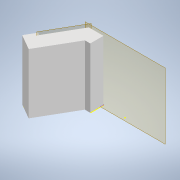
# Autodesk Inventor part: Задние_кресла
Saved by Autodesk Inventor 2021.2 (Build 252289000, 289)
## iProperties
Created: 2021-10-13
Part Number: Задние_кресла
Material: Типовые
Document SubType Name: Modeling
Designer: Surflay
Density: 1 g/cm^3
Appearance: По умолчанию
Author: Surflay
Autodesk Inventor part; units mm, degrees
ref_plane "YZ Plane" through (0, 0, 0) normal (1, 0, 0) x (0, 1, 0)
ref_plane "XZ Plane" through (0, 0, 0) normal (0, 1, 0) x (-1, 0, 0)
ref_plane "XY Plane" through (0, 0, 0) normal (0, 0, 1) x (1, 0, 0)
ref_plane "РабПлоскость1" through (0, 0, 0) normal (0, 0, 1) x (1, 0, 0)
sketch "Эскиз1" plane through (0, 0, 0) normal (0, 0, 1) x (1, 0, 0)
  line L0 (-185, -102) -> (-185, 102) projected
  line L1 (-123.5, -102) -> (-185, -102) projected
  line L2 (-123.5, 102) -> (-123.5, -102) projected
  line L3 (-185, 102) -> (-123.5, 102) projected
  line L4 (-123.5, 102) -> (-123.5, -102) projected
  line L5 (-123.5, -102) -> (123.5, -102) projected
  line L6 (123.5, -102) -> (123.5, -100.4305) projected
  line L7 (123.5, -100.4305) -> (123.5, 102) projected
  line L8 (123.5, 102) -> (-123.5, 102) projected
  line L9 (-123.5, -102) -> (-73.5, -102)
  line L10 (-73.5, -102) -> (-73.5, 102)
  line L11 (-73.5, 102) -> (-123.5, 102)
  line L12 (-123.5, 102) -> (-123.5, -102)
  point P0 (0, 0)
  dimension "d0" = 50
  constraints: 8 end point, 2 parallel, 1 horizontal, 1 perpendicular, 1 point on line
  measures "d0" distance of L11.end L10.end
extrude "Выдавливание1" add sketch "Эскиз1" along normal blind 45 contours L2 L8 L10 L5
ref_plane "РабПлоскость2" through (-154.25, 0, 53.2606) normal (0.866, 0, 0.5) x (0, 1, 0)
sketch "Эскиз2" plane through (-154.25, 0, 53.2606) normal (0.866, 0, 0.5) x (0, 1, 0)
  line L0 (-102, 61.5) -> (102, 61.5) projected
  line L1 (-102, -61.5) -> (-102, 61.5) projected
  line L2 (102, -61.5) -> (-102, -61.5) projected
  line L3 (102, 61.5) -> (102, -61.5) projected
  line L4 (102, -61.5) -> (-102, -61.5) projected
  line L5 (-102, -61.5) -> (-102, -185) projected
  line L6 (-102, -185) -> (-100.4305, -185) projected
  line L7 (-100.4305, -185) -> (102, -185) projected
  line L8 (102, -185) -> (102, -61.5) projected
  line L9 (102, -61.5) -> (-102, -61.5) projected
  line L10 (-102, -61.5) -> (-102, -22.5289) projected
  line L11 (102, -22.5289) -> (-102, -22.5289) projected
  line L12 (102, -61.5) -> (102, -22.5289) projected
  line L13 (-102, -61.5) -> (102, -61.5)
  line L14 (102, -61.5) -> (102, 61.5)
  line L15 (102, 61.5) -> (-102, 61.5)
  line L16 (-102, 61.5) -> (-102, -61.5)
  line L17 (-102, 61.5) -> (102, 61.5)
  line L18 (102, 61.5) -> (102, 101.5)
  line L19 (102, 101.5) -> (-102, 101.5)
  line L20 (-102, 101.5) -> (-102, 61.5)
  point P0 (0, -123.25)
  dimension "d3" = 40
  constraints: 16 end point, 4 parallel, 2 horizontal, 2 perpendicular, 1 point on line
  measures "d3" distance of L18.end L17.end
extrude "Выдавливание2" add sketch "Эскиз2" along normal blind 50 contours L20 L19 L18 L0 | L0 L3 L11 L1 | L11 L3 L2 L1
sketch "Эскиз3" plane through (-73.5, -102, 0) normal (0, -1, 0) x (1, 0, 0)
  line L0 (-108.6908, 129.6314) -> (-111.6772, 121.8416)
  line L1 (-105.4631, 130.9264) -> (-108.6908, 129.6314)
  line L2 (-103.4661, 130.9653) -> (-105.4631, 130.9264)
  line L3 (-100.0404, 130.4564) -> (-103.4661, 130.9653)
  line L4 (-95.5925, 122.215) -> (-100.0404, 130.4564)
  line L5 (-93.9034, 112.6939) -> (-95.5925, 122.215)
  line L6 (-111.6772, 121.8416) -> (-110.616, 112.412)
  line L7 (-111.3059, 112.062) -> (-115.4641, 110.9539)
  line L8 (-104.8347, 111.7616) -> (-111.3059, 112.062)
  line L9 (-99.8505, 111.497) -> (-104.8347, 111.7616)
  line L10 (-115.4641, 110.9539) -> (-114.6124, 106.4901)
  line L11 (-93.7292, 100.7609) -> (-99.8505, 111.497)
  line L12 (-72.7658, 69.3465) -> (-93.7292, 100.7609)
  line L13 (-63.261, 43.1561) -> (-72.1915, 66.6367)
  line L14 (-57.7493, 27.3924) -> (-63.261, 43.1561)
  line L15 (-42.1622, 38.0832) -> (-61.3633, 33.05)
  line L16 (-3.3347, 28.5944) -> (-17.584, 40.2262)
  line L17 (-2.0035, -1.7748) -> (-3.3347, 28.5944)
  line L18 (-42.1622, 38.0832) -> (-17.584, 40.2262)
  line L19 (-111.2907, 111.9869) -> (-115.4518, 110.8898)
  line L20 (-115.4478, 110.4521) -> (-115.4518, 110.8898)
  line L21 (-94.9926, 106.7102) -> (-93.9034, 112.6939)
  line L22 (-97.6358, 105.6373) -> (-94.9926, 106.7102)
  line L23 (-114.6124, 106.4901) -> (-115.4518, 110.8898)
  line L24 (-111.2907, 111.9869) -> (-110.616, 112.412)
  line L25 (-111.6772, 121.8416) -> (-108.6022, 131.2469)
  line L26 (-108.6022, 131.2469) -> (-105.4955, 132.5857)
  line L27 (-105.4955, 132.5857) -> (-103.375, 132.6268)
  line L28 (-103.375, 132.6268) -> (-99.8731, 132.148)
  line L29 (-99.8731, 132.148) -> (-95.5925, 122.215)
  line L30 (-95.5925, 122.215) -> (-93.9034, 112.6939)
  line L31 (-94.9926, 106.7102) -> (-93.9034, 112.6939)
  line L32 (-94.9926, 106.7102) -> (-96.7212, 106.0085)
  line L33 (-96.7212, 106.0085) -> (-93.7292, 100.7609)
  line L34 (-93.7292, 100.7609) -> (-72.7658, 69.3465)
  line L35 (-72.7658, 69.3465) -> (-59.8648, 33.4429)
  line L36 (-59.8648, 33.4429) -> (-42.1622, 38.0832)
  line L37 (-42.1622, 38.0832) -> (-17.584, 40.2262)
  line L38 (-17.584, 40.2262) -> (-3.3347, 28.5944)
  line L39 (-3.3347, 28.5944) -> (-3.3082, 27.9912)
  line L40 (-2.1491, 1.5473) -> (-2.1491, 0.2174)
  line L41 (-2.1491, 0.2174) -> (-50.02, 0.2174)
  line L42 (-114.6455, 106.6636) -> (-115.4518, 110.8898)
  line L43 (-50, 0) -> (0, 0) projected
  line L44 (-50, 0) -> (-111.4821, 106.4901)
  line L45 (-50, 0) -> (-131.5, 141.1621) projected
  line L46 (-111.4821, 106.4901) -> (-114.6124, 106.4901)
  line L47 (0, 0) -> (0, 45) projected
  line L48 (0, 1.5473) -> (-1.7253, 27.8714)
  line L49 (0, 1.5473) -> (-8.568, 1.5473)
  line L50 (-1.7253, 27.8714) -> (-6.6021, 27.8714)
  line L51 (0, 1.5473) -> (0, 27.8714)
  line L52 (0, 0) -> (0, 45) projected
  line L53 (0, 27.8714) -> (-1.7253, 27.8714)
  point P0 (73.5, 0)
  point P1 (-3.303, 27.8714)
  point P2 (-2.0813, 0)
  point P3 (-2.1491, 1.5473)
  point P4 (0, 27.8714)
  constraints: 100 end point, 10 point on line, 7 collinear, 3 horizontal, 3 perpendicular, 1 vertical
sketch "Эскиз4" plane through (-154.25, 0, 53.2606) normal (-0.866, 0, -0.5) x (-0.5, 0, 0.866)
  line L0 (111.8349, 102) -> (121.8349, 82) projected
  line L1 (111.8349, 102) -> (61.5, 102) projected
  line L2 (61.5, -102) -> (61.5, 102) projected
  line L3 (61.5, -102) -> (111.8349, -102) projected
  line L4 (121.8349, -82) -> (111.8349, -102) projected
  line L5 (121.8349, -82) -> (121.8349, 82) projected
  line L6 (101.5, 102) -> (101.5, -102) projected
  line L7 (-61.5, 102) -> (101.5, 102) projected
  line L8 (-61.5, 102) -> (-61.5, -102) projected
  line L9 (101.5, -102) -> (-61.5, -102) projected
  line L10 (101.5, 102) -> (101.5, -102) projected
  line L11 (101.5, 102) -> (61.5, 102)
  line L12 (61.5, 102) -> (61.5, -102)
  line L13 (61.5, -102) -> (101.5, -102)
  line L14 (101.5, -102) -> (101.5, 102)
  point P0 (-123.25, 0)
  point P1 (101.5, -102)
  constraints: 8 end point, 2 parallel, 1 horizontal, 1 perpendicular
extrude "Выдавливание3" add sketch "Эскиз4" along normal blind 10 contours L6 L3 L2 L1
extrude "Выдавливание4" cut sketch "Эскиз3" against normal through all contours L1 L2 L3 L4 L5 L21 L22 L11 L9 L8 L24 L6 L0 | L0 L25 L26 L27 L28 L29 L4 L3 L2 L1 | L8 L9 L11 L12 L35 L15 L18 L16 L17 L43 L44 L45 L19 L24 | L45 L46 L10 L19 | L17 L50 L48 L49 | L48 L53 L47 keep common part
sketch "Эскиз5" plane through (-73.5, -102, 27.8714) normal (1, 0, 0) x (0, 0, -1)
  line L0 (0, 0) -> (0, 204) construction
  line L1 (0, 0) -> (0, 204) construction
  line L2 (-0.723, 204) -> (-12.3548, 204) projected
  line L3 (-12.3548, 0) -> (-12.3548, 204) construction
  line L4 (-12.3548, 0) -> (-0.723, 0) projected
  line L5 (-0.723, 0) -> (-0.723, 204) construction
  line L6 (-12.3548, 204) -> (-10.2118, 204) projected
  line L7 (-10.2118, 0) -> (-10.2118, 204) construction
  line L8 (-10.2118, 0) -> (-12.3548, 0) projected
  line L9 (-12.3548, 0) -> (-12.3548, 204) construction
  line L10 (-10.2118, 204) -> (-5.5715, 204) projected
  line L11 (-5.5715, 0) -> (-5.5715, 204) construction
  line L12 (-5.5715, 0) -> (-10.2118, 0) projected
  line L13 (-10.2118, 0) -> (-10.2118, 204) construction
  line L14 (-5.5715, 204) -> (-41.4751, 204) projected
  line L15 (-41.4751, 0) -> (-41.4751, 204) construction
  line L16 (-41.4751, 0) -> (-5.5715, 0) projected
  line L17 (-5.5715, 0) -> (-5.5715, 204) construction
  line L18 (-41.4751, 204) -> (-72.8895, 204) projected
  line L19 (-72.8895, 0) -> (-72.8895, 204) construction
  line L20 (-72.8895, 0) -> (-41.4751, 0) projected
  line L21 (-41.4751, 0) -> (-41.4751, 204) construction
  line L22 (-72.8895, 204) -> (-78.1371, 204) projected
  line L23 (-78.1371, 0) -> (-78.1371, 204) construction
  line L24 (-78.1371, 0) -> (-72.8895, 0) projected
  line L25 (-72.8895, 0) -> (-72.8895, 204) construction
  line L26 (-84.8225, 204) -> (-94.3436, 204) projected
  line L27 (-94.3436, 0) -> (-94.3436, 204) construction
  line L28 (-94.3436, 0) -> (-84.8225, 0) projected
  line L29 (-84.8225, 0) -> (-84.8225, 204) construction
  line L30 (-94.3436, 204) -> (-104.2766, 204) projected
  line L31 (-104.2766, 0) -> (-104.2766, 204) construction
  line L32 (-104.2766, 0) -> (-94.3436, 0) projected
  line L33 (-94.3436, 0) -> (-94.3436, 204) construction
  line L34 (-104.2766, 204) -> (-104.7554, 204) projected
  line L35 (-104.7554, 0) -> (-104.7554, 204) construction
  line L36 (-104.7554, 0) -> (-104.2766, 0) projected
  line L37 (-104.2766, 0) -> (-104.2766, 204) construction
  line L38 (-79.9479, 207.7487) -> (-84.8032, 203.5165)
  line L39 (-84.8032, 203.5165) -> (-84.8032, 189.9966)
  line L40 (-84.8032, 189.9966) -> (-84.8032, 189.4946)
  line L41 (-84.8032, 189.4946) -> (-86.5261, 189.6155)
  line L42 (-86.5261, 189.6155) -> (-95.9527, 185.6405)
  line L43 (-95.9527, 185.6405) -> (-104.2286, 180.7662)
  line L44 (-104.2286, 180.7662) -> (-105.6998, 178.2579)
  line L45 (-105.6998, 178.2579) -> (-105.6998, 155.6836)
  line L46 (-105.6998, 155.6836) -> (-104.2286, 152.809)
  line L47 (-104.2286, 152.809) -> (-95.9527, 147.0033)
  line L48 (-95.9527, 147.0033) -> (-86.5261, 141.9023)
  line L49 (-86.5261, 141.9023) -> (-83.8361, 141.9023)
  line L50 (-83.8361, 141.9023) -> (-83.8361, 126.2664)
  line L51 (-83.8361, 126.2664) -> (-86.5261, 126.2664)
  line L52 (-86.5261, 126.2664) -> (-95.9527, 121.7556)
  line L53 (-95.9527, 121.7556) -> (-104.2286, 116.4608)
  line L54 (-104.2286, 116.4608) -> (-105.6998, 113.4827)
  line L55 (-105.6998, 113.4827) -> (-105.6998, 91.4649)
  line L56 (-105.6998, 91.4649) -> (-104.2286, 88.3904)
  line L57 (-104.2286, 88.3904) -> (-95.9527, 83.0098)
  line L58 (-95.9527, 83.0098) -> (-86.5261, 78.5722)
  line L59 (-86.5261, 78.5722) -> (-83.8361, 78.5722)
  line L60 (-83.8361, 78.5722) -> (-83.8361, 78.5722)
  line L61 (-95.9527, 58.8646) -> (-104.2286, 52.9602)
  line L62 (-104.2286, 52.9602) -> (-105.6998, 49.835)
  line L63 (-105.6998, 49.835) -> (-105.6998, 27.8897)
  line L64 (-105.6998, 27.8897) -> (-104.2949, 24.9539)
  line L65 (-104.2949, 24.9539) -> (-95.9527, 20.1778)
  line L66 (-95.9527, 20.1778) -> (-86.4193, 16.1382)
  line L67 (-86.4193, 16.1382) -> (-83.8361, 16.357)
  line L68 (-83.8361, 16.357) -> (-83.8361, 16.357)
  line L69 (-95.9527, 58.8646) -> (-86.3102, 63.8843)
  line L70 (-86.3102, 63.8843) -> (-83.8361, 63.9034)
  line L71 (-83.8361, 63.9034) -> (-83.8361, 78.5722)
  line L72 (-79.9479, 207.7487) -> (-66.9821, 209.4381)
  line L73 (-66.9821, 209.4381) -> (-41.1997, 209.4381)
  line L74 (-41.1997, 209.4381) -> (-14.9178, 205.9692)
  line L75 (-14.9178, 205.9692) -> (-13.7255, 207.2288)
  line L76 (-13.7255, 207.2288) -> (-5.445, 207.1235)
  line L77 (-5.445, 207.1235) -> (19.6874, 206.8037)
  line L78 (19.6874, 206.8037) -> (23.2689, 204.6715)
  line L79 (23.2689, 204.6715) -> (23.2603, 204)
  line L80 (27.8714, 204) -> (27.8714, 5)
  line L81 (27.8714, 5) -> (22.8162, 5)
  line L82 (22.8162, 5) -> (22.8162, -0.7369)
  line L83 (22.8162, -0.7369) -> (19.0771, -2.2962)
  line L84 (19.0771, -2.2962) -> (-14.3617, -2.5553)
  line L85 (-14.3617, -2.5553) -> (-18.3756, 1.978)
  line L86 (-18.3756, 1.978) -> (-18.3756, 6.9468)
  line L87 (-18.3756, 6.9468) -> (-14.4728, 11.7843)
  line L88 (-14.4728, 11.7843) -> (-7.2373, 11.8403)
  line L89 (-7.2373, 11.8403) -> (-7.2373, 192.6157)
  line L90 (-7.2373, 192.6157) -> (-13.7255, 192.8411)
  line L91 (-13.7255, 192.8411) -> (-17.7394, 197.6844)
  line L92 (-17.7394, 197.6844) -> (-17.7394, 202.5296)
  line L93 (-17.7394, 202.5296) -> (-13.7255, 207.2288)
  line L94 (-14.3617, -2.5553) -> (-16.3687, -0.2886)
  line L95 (-16.3687, -0.2886) -> (-40.0618, -4.056)
  line L96 (-40.0618, -4.056) -> (-41.8359, -4.0697)
  line L97 (-41.8359, -4.0697) -> (-67.6183, -4.0697)
  line L98 (-67.6183, -4.0697) -> (-77.5196, -2.7629)
  line L99 (-77.5196, -2.7629) -> (-80.7406, -2.2382)
  line L100 (-80.7406, -2.2382) -> (-85.215, 1.6269)
  line L101 (-85.215, 1.6269) -> (-85.215, 9.2117)
  line L102 (-85.215, 9.2117) -> (-85.215, 16.2402)
  line L103 (27.8714, 0) -> (27.8714, 204) projected
  line L104 (27.8714, 204) -> (27.8714, 0) projected
  line L105 (27.8714, 199) -> (23.2603, 199)
  line L106 (23.2603, 199) -> (23.2603, 204)
  line L107 (29.4197, 204) -> (-28.798, 204)
  line L108 (-78.6497, 0) -> (27.8714, 0) projected
  line L109 (-12.3548, 11.8007) -> (-12.3548, 192.7935)
  point P0 (27.8714, 102)
  point P1 (22.8162, 0)
  point P2 (-16.4835, 204)
  point P3 (-104.2766, 180.6842)
  point P4 (-104.2766, 152.9028)
  point P5 (-104.2766, 116.3636)
  point P6 (-104.2766, 88.4908)
  point P7 (-104.2766, 52.8582)
  point P8 (-104.2766, 24.9434)
  point P9 (-84.8225, 16.2734)
  point P10 (-84.8225, 1.2878)
  point P11 (-16.6242, 0)
  point P12 (-94.3436, 82.2523)
  point P13 (-94.3436, 59.7022)
  point P14 (-94.3436, 146.1326)
  point P15 (-94.3436, 122.5256)
  point P16 (-13.7255, 207.2288)
  point P17 (-104.7554, 153.8384)
  point P18 (-104.7554, 115.3943)
  point P19 (-104.7554, 89.4914)
  point P20 (-104.7554, 51.841)
  point P21 (-104.7554, 25.9162)
  point P22 (-104.2766, 24.9434)
  point P23 (-104.2766, 180.6842)
  point P24 (-104.7554, 179.8679)
  point P25 (-104.2766, 152.9028)
  point P26 (-104.2766, 116.3636)
  point P27 (-104.2766, 88.4908)
  point P28 (-104.2766, 52.8582)
  dimension "d10" = 204
  dimension "d12" = 5
  dimension "d13" = 5
  constraints: 136 end point, 18 point on line, 14 perpendicular, 4 parallel, 3 vertical, 1 horizontal, 1 midpoint, 4 other
  measures "d10" distance of L103.start L80.start
  measures "d13" distance of the line from the sketch origin of L81
sketch "Эскиз7" plane through (-73.5, -102, 27.8714) normal (1, 0, 0) x (0, 0, -1)
  line L0 (-14.4728, 11.7843) -> (-7.2373, 11.8403) projected
  line L1 (-7.2373, 11.8403) -> (-7.2373, 192.6583)
  line L2 (-5.5715, 0) -> (-5.5715, 204) projected
  line L3 (-7.2373, 192.6583) -> (-12.3548, 192.8032)
  line L4 (-12.3548, 0) -> (-12.3548, 204) projected
  line L5 (-12.3548, 192.8032) -> (-12.3548, 11.8007)
  line L6 (-12.3548, 11.8007) -> (-7.2373, 11.8403)
  line L7 (-7.2373, 192.6583) -> (-12.3548, 192.8032)
  line L8 (-7.2373, 11.8403) -> (-5.5715, 11.8403)
  line L9 (-5.5715, 192.6583) -> (-7.2373, 192.6583)
  line L10 (-5.5715, 11.8403) -> (-5.5715, 192.6583)
  point P0 (27.8714, 102)
  constraints: 16 end point, 4 point on line, 3 parallel, 2 perpendicular, 1 collinear
extrude "Выдавливание6" cut sketch "Эскиз7" against normal up to surface surface through (-146.2658, -102, 69.3465) normal (0.9411, 0, 0.3382)
extrude "Выдавливание7" cut sketch "Эскиз5" against normal up to surface contours L107 L106 L105 L80 L81 L82 L108 L4 L16 L85 L86 L87 L88 L89 L90 L91 L92 L93 L14 L2 | L2 L14 L93 L76 L77 L78 L79 L107 | L93 L92 L91 L90 L109 L88 L87 L86 L85 L95 L96 L97 L98 L99 L100 L101 L102 L67 L66 L65 L64 L63 L62 L61 L69 L70 L71 L59 L58 L57 L56 L55 L54 L53 L52 L51 L50 L49 L48 L47 L46 L45 L44 L43 L42 L41 L40 L39 L38 L72 L73 L74 L75 | L82 L83 L84 L85 L16 L4 L108 | L90 L89 L88 L109 surface through (-164.25, 0, 70.5811) normal (0.866, 0, 0.5) keep common part
